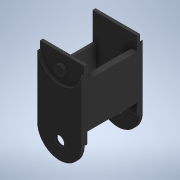
# Autodesk Inventor part: Eslabon cadena portacable
Saved by Autodesk Inventor 2020 (Build 240168000, 168)
## iProperties
Created: 2020-07-05
Part Number: Eslabon cadena portacable
Material: Genérico
Document SubType Name: Modeling
Designer: Pipi
Density: 1 g/cm^3
Appearance: Goma - Negro
Author: Pipi
Autodesk Inventor part; units mm, degrees
ref_plane "YZ Plane" through (0, 0, 0) normal (1, 0, 0) x (0, 1, 0)
ref_plane "XZ Plane" through (0, 0, 0) normal (0, 1, 0) x (-1, 0, 0)
ref_plane "XY Plane" through (0, 0, 0) normal (0, 0, 1) x (1, 0, 0)
sketch "Boceto1" plane through (0, 0, 0) normal (0, 1, 0) x (-1, 0, 0)
  line L0 (10.3005, 0.2018) -> (-1.6995, 0.2018)
  line L1 (-1.6995, 0.2018) -> (-1.6995, 18.2018)
  line L2 (-1.6995, 18.2018) -> (10.3005, 18.2018)
  line L3 (12.3005, 20.2018) -> (-3.6995, 20.2018)
  line L4 (-3.6995, 20.2018) -> (-3.6995, -1.7982)
  line L5 (-3.6995, -1.7982) -> (12.3005, -1.7982)
  line L6 (10.3005, 18.2018) -> (12.3005, 18.2018)
  line L7 (10.3005, 0.2018) -> (12.3005, 0.2018)
  line L8 (12.3005, -1.7982) -> (12.3005, 0.2018)
  line L9 (12.3005, 18.2018) -> (12.3005, 20.2018)
  point P0 (0, 0)
  dimension "d0" = 18
  dimension "d1" = 12
  constraints: 20 end point, 10 perpendicular, 2 other
  measures "d0" distance of L2.end L0.start
  measures "d1" distance of L0.start L0.end
extrude "Extrusión1" add sketch "Boceto1" along normal blind 25
sketch "Boceto2" plane through (-12.3005, 0, 20.2018) normal (0, 0, 1) x (1, 0, 0)
  line L0 (16, 0) -> (16, 25) projected
  line L1 (0, 0) -> (14, 0) projected
  arc A0 (0, 0) -> (16, 0) centre (8, 0) ccw
  line L2 (0, 0) -> (16, 0)
  constraints: 2 end point, 2 point on circle, 1 centre point, 1 horizontal, 1 tangent
sketch "Boceto3" plane through (3.6995, 0, -1.7982) normal (0, 0, -1) x (-1, 0, 0)
  line L0 (0, 0) -> (0, 25) projected
  line L1 (16, 0) -> (16, 25) projected
  arc A0 (0, 0) -> (16, 0) centre (8, -0.0367) ccw
  line L2 (16, 0) -> (0, 0)
  line L3 (16, 0) -> (2, 0) projected
  point P0 (3.6995, 0)
  constraints: 2 end point, 2 point on circle, 1 centre point, 1 collinear
extrude "Extrusión2" add sketch "Boceto3" against normal blind 1
extrude "Extrusión3" add sketch "Boceto2" against normal blind 1
sketch "Boceto5" plane through (3.6995, 25, -1.7982) normal (0, 0, -1) x (-1, 0, 0)
  line L0 (0, 0) -> (16, 0) projected
  line L1 (16, -25) -> (16, 0) projected
  line L2 (16, 0) -> (0, 0)
  line L3 (16, 0) -> (16, -1.5)
  line L4 (16, 0) -> (0, 0)
  line L5 (0, -25) -> (0, 0) projected
  line L6 (0, 0) -> (0, -1.5)
  arc A0 (0.0504, -2.3965) -> (15.9464, -2.4245) centre (8, -1.5) ccw
  line L7 (15.9464, -2.4245) -> (15.9666, -2.3645)
  arc A1 (16, -2.3216) -> (15.9666, -2.3645) centre (16.045, -2.3909) ccw
  line L8 (0.0504, -2.3965) -> (0.0316, -2.3763)
  arc A2 (0.0316, -2.3763) -> (0, -2.3536) centre (-0.0406, -2.4434) ccw
  line L9 (16, -2.3216) -> (16, -1.5)
  line L10 (0, -1.5) -> (0, -2.3536)
  point P0 (3.6995, -25)
  dimension "d13" = 1.5
  constraints: 16 end point, 6 point on circle, 4 collinear, 4 point on line, 4 tangent, 3 centre point
  measures "d13" distance of L0.end L3.end
sketch "Boceto6" plane through (-12.3005, 25, 20.2018) normal (0, 0, 1) x (1, 0, 0)
  line L0 (16, 0) -> (0, 0) projected
  line L1 (16, -25) -> (16, 0) projected
  line L2 (0, 0) -> (16, 0)
  line L3 (0, 0) -> (0, -1.5)
  line L4 (0, -25) -> (0, 0) projected
  arc A0 (0.0942, -2.7242) -> (15.9182, -2.6413) centre (8, -1.5) ccw
  line L5 (16, -1.5) -> (16, 0)
  line L6 (15.9182, -2.6413) -> (15.9286, -2.6198)
  arc A1 (16, -2.5333) -> (15.9286, -2.6198) centre (16.1434, -2.7242) ccw
  line L7 (0.0942, -2.7242) -> (0.0677, -2.6601)
  arc A2 (0.0677, -2.6601) -> (0, -2.5946) centre (-0.0415, -2.7053) ccw
  line L8 (16, -2.5333) -> (16, 0)
  line L9 (0, -2.5946) -> (0, 0)
  point P0 (12.3005, -25)
  dimension "d10" = 1.5
  constraints: 14 end point, 6 point on circle, 4 point on line, 3 centre point, 3 collinear, 3 tangent, 1 horizontal
  measures "d10" distance of L0.end L3.end
extrude "Extrusión4" cut sketch "Boceto6" against normal blind 1
extrude "Extrusión5" cut sketch "Boceto5" against normal blind 1
sketch "Boceto8" plane through (-4.3005, -0.0367, -1.7982) normal (0, 0, -1) x (-1, 0, 0)
  circle A0 centre (0.1375, 20.0367) radius 1.75
  circle A1 centre (0.0632, -1.9632) radius 1.75
  line L0 (-8, 25.0367) -> (8, 25.0367) projected
  point P0 (-4.3005, 0.0367)
  dimension "d19" = 3.5
  dimension "d20" = 3.5
  dimension "d21" = 22
  dimension "d22" = 5
  constraints: 2 centre point
  measures "d19" diameter of A0
  measures "d20" diameter of A1
  measures "d21" distance of A1.centre A0.centre
  measures "d22" distance from line of L0 A0.centre
extrude "Extrusión6" add sketch "Boceto8" against normal blind 1 contours A0
extrude "Extrusión7" cut sketch "Boceto8" against normal blind 30 contours A1
sketch "Boceto9" plane through (-12.3005, 25, 19.2018) normal (0, 0, 1) x (1, 0, 0)
  circle A0 centre (7.8625, -5) radius 1.75 projected
  circle A1 centre (7.8625, -5) radius 1.75
  point P0 (12.3005, -25)
  constraints: 1 centre point, 1 coincident
extrude "Extrusión8" add sketch "Boceto9" along normal blind 1
sketch "Boceto10" plane through (-12.3005, 0, 0.2018) normal (-1, 0, 0) x (0, 0, 1)
  line L0 (-2, 0) -> (-2, 22.6784) projected
  line L1 (20, 0) -> (20, 22.4054) projected
  line L2 (0, 14.992) -> (18, 14.992)
  line L3 (0, 6.992) -> (18, 6.992)
  line L4 (0, 0) -> (0, 25) projected
  line L5 (0, 6.992) -> (0, 14.992)
  line L6 (18, 0) -> (18, 25) projected
  line L7 (18, 6.992) -> (18, 14.992)
  point P0 (-0.2018, 0)
  dimension "d32" = 8
  constraints: 8 end point, 4 point on line, 1 perpendicular
  measures "d32" distance between parallel lines of L2 L3
extrude "Extrusión9" add sketch "Boceto10" against normal blind 1
sketch "Boceto11" plane through (3.6995, 0, -0.7982) normal (1, 0, 0) x (0, 0, -1)
  point P0 (-0.7982, 0)
sketch "Boceto12" plane through (1.6995, 0, 0.2018) normal (-1, 0, 0) x (0, 0, 1)
  line L0 (0, 14.992) -> (0, 25) projected
  line L1 (0, 25) -> (0, 20)
  line L2 (0, 20) -> (18, 20)
  line L3 (18, 14.992) -> (18, 25) projected
  line L4 (18, 25) -> (0, 25)
  line L5 (19, 25) -> (-1, 25) projected
  line L6 (18, 25) -> (18, 20)
  line L7 (-1, 0) -> (0, 0) projected
  line L8 (0, 0) -> (0, 4)
  line L9 (0, 0) -> (0, 25) projected
  line L10 (0, 4) -> (18, 4)
  line L11 (18, 0) -> (18, 25) projected
  line L12 (0, 0) -> (18, 0) projected
  line L13 (18, 4) -> (18, 0)
  line L14 (18, 0) -> (0, 0)
  point P0 (-0.2018, 0)
  dimension "d35" = 5
  dimension "d36" = 4
  constraints: 16 end point, 4 point on line, 3 perpendicular, 2 collinear, 1 vertical
  measures "d35" distance of L0.end L1.end
  measures "d36" distance of L7.end L8.end
extrude "Extrusión10" cut sketch "Boceto12" against normal blind 2 contours L0 L4 L3 L2 | L10 L11 L12 L8
